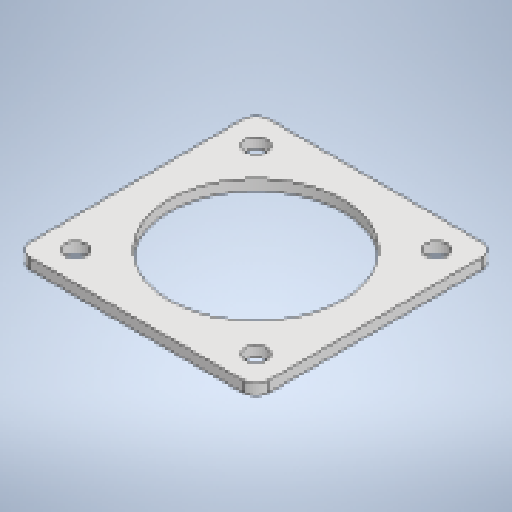
# Autodesk Inventor part: NDM-VOS 162 harrow plate 5
Saved by Autodesk Inventor 2025.1 (Build 291241020, 241B)
## iProperties
Created: 2024-11-03
Part Number: NDM-VOS 162 harrow plate 5
Material: Stainless Steel
Document SubType Name: Sheet Metal
Designer: user
Mass: 280.619 g
Surface Area: 364.406 cm^2
Volume: 35.0774 cm^3
Density: 8 g/cm^3
Sheet Metal Rule: AISI304 3mm Die 32
Sheet Metal Width: 0,000 mm
Sheet Metal Length: 0,000 mm
Sheet Metal Area: 0,000 mm^2
Appearance: Default
Author: admin
Гриндер_отступ_отврс_корпуса: 25.000 mm
Гриндер_диам_отврс_корпуса: 13.000 mm
Гриндер_проходная_ширина: 320.000 mm
Гриндер_проходная_длина: 320.000 mm
Гриндер_высота: 200.000 mm
Гриндер_размер_фланца: 40.000 mm
Гриндер_Валы_между_центрами: 150.000 mm
Autodesk Inventor part; units mm, degrees
ref_plane "YZ Plane" through (0, 0, 0) normal (1, 0, 0) x (0, 1, 0)
ref_plane "XZ Plane" through (0, 0, 0) normal (0, 1, 0) x (-1, 0, 0)
ref_plane "XY Plane" through (0, 0, 0) normal (0, 0, 1) x (1, 0, 0)
sketch "Sketch1" plane through (0, 0, 0) normal (0, 0, 1) x (1, 0, 0)
  line L0 (-200, 100) -> (200, 100)
  line L1 (200, 100) -> (200, -100)
  line L2 (200, -100) -> (-200, -100)
  line L3 (-200, -100) -> (-200, 100)
  line L4 (-200, 100) -> (200, -100) construction
  line L5 (200, 100) -> (-200, -100) construction
  point P0 (0, 0)
  point P1 (0, 0)
  point P2 (0, 0)
  dimension "d25" = 400
  dimension "d26" = 200
  measures "d25" distance of L1.end L2.end
  measures "d26" distance of L0.end L1.end
extrude "Plate1" add sketch "Sketch1" along normal blind 5
sketch "Sketch5" plane through (-195, -100, 0) normal (-1, 0, 0) x (0, -1, 0)
  line L0 (-200, 0) -> (0, 0)
  line L1 (0, 0) -> (0, 50)
  line L2 (0, 50) -> (-200, 50)
  line L3 (-200, 50) -> (-200, 0)
  constraints: 6 end point, 1 horizontal, 1 perpendicular, 1 vertical
edge flange "Flange2" height 50 angle 90 thickness 5 bend radius 5 thickness toward (-1, 0, 0) relief round relief width 5 relief depth 2.5 corner gap 5 corner form 0 edges at (-200, 0, 5) (200, 0, 5) (0, 100, 5) (0, -100, 5) wall of the first edge with corners at (-195, 100, 0) (-195, -100, 0) (-195, -100, 50) (-195, 100, 50)
bend "Bend2"
corner "Corner2"
sketch "Sketch6" plane through (0, 0, 5) normal (0, 0, 1) x (1, 0, 0)
  circle A0 centre (-75, 0) radius 16
  circle A1 centre (75, 0) radius 16
  line L0 (0, 0) -> (0, 55.0725) construction
  circle A2 centre (33.5, 41.5) radius 5
  circle A3 centre (116.5, 41.5) radius 5
  circle A4 centre (116.5, -41.5) radius 5
  circle A5 centre (33.5, -41.5) radius 5
  line L1 (75, 0) -> (-75, 0)
  line L2 (75, 0) -> (75, -40.8866)
  circle A6 centre (-33.5, 41.5) radius 5
  circle A7 centre (-116.5, 41.5) radius 5
  circle A8 centre (-116.5, -41.5) radius 5
  circle A9 centre (-33.5, -41.5) radius 5
  point P0 (-75, -40.8866)
  dimension "d37" = 32
  dimension "d38" = 150
  dimension "d55" = 10
  dimension "d56" = 83
  dimension "d57" = 83
  constraints: 10 centre point, 8 symmetric about line, 6 end point, 3 equal radius, 3 horizontal alignment, 2 vertical, 2 vertical alignment, 1 horizontal, 5 other
  measures "d37" diameter of A0
  measures "d38" distance of L1.start L1.end
  measures "d55" diameter of A3
  measures "d56" distance of A3.centre A2.centre
  measures "d57" distance of A4.centre A3.centre
extrude "Cut1" cut sketch "Sketch6" against normal blind 5
sketch "Sketch7" plane through (-194.2929, 100, 10) normal (0, 1, 0) x (1, 0, 0)
  circle A0 centre (194.2929, -20) radius 6.5
  line L0 (5, 5) -> (383.5858, 5) projected
  line L1 (383.5858, 5) -> (384.2929, 5) projected
  line L2 (384.2929, 5) -> (383.5858, 5) projected
  line L3 (383.5858, 5) -> (5, 5) projected
  line L4 (5, 5) -> (4.2929, 5) projected
  line L5 (4.2929, 5) -> (5, 5) projected
  point P0 (194.2929, 10)
  dimension "d41" = 13
  dimension "d42" = 25
  constraints: 1 centre point, 1 vertical alignment
  measures "d41" diameter of A0
  measures "d42" distance from line of A0.centre L0
extrude "Extrusion2" cut sketch "Sketch7" against normal through all
pattern_linear "Rectangular Pattern1" count 3 spacing 160 along (-1, 0, 0) of "Extrusion2" first direction both ways yes
sketch "Sketch8" plane through (0, 0, 0) normal (1, 0, 0) x (0, 1, 0)
  line L0 (-94.2929, 50) -> (94.2929, 50) projected
  circle A0 centre (0, 30) radius 6.5
  line L1 (89.2929, 5) -> (-89.2929, 5) projected
  point P0 (0, 0)
  dimension "d48" = 13
  dimension "d49" = 25
  constraints: 1 centre point, 1 vertical alignment
  measures "d48" diameter of A0
  measures "d49" distance from line of L1 A0.centre
extrude "Extrusion3" cut sketch "Sketch8" along normal through all both and the other way through all
pattern_linear "Rectangular Pattern2" count 3 spacing 70 along (0, 1, 0) of "Extrusion3" first direction both ways yes
sketch "Sketch9" plane through (0, 0, 0) normal (0, 0, 1) x (1, 0, 0)
  line L0 (-233.1694, -164.5287) -> (298.5547, -164.5287)
  line L1 (298.5547, -164.5287) -> (298.5547, 258.31)
  line L2 (298.5547, 258.31) -> (-233.1694, 258.31)
  line L3 (-233.1694, 258.31) -> (-233.1694, -164.5287)
  circle A0 centre (-75, 0) radius 16 projected
  line L4 (-130, -55) -> (-20, -55)
  line L5 (-20, -55) -> (-20, 55)
  line L6 (-20, 55) -> (-130, 55)
  line L7 (-130, 55) -> (-130, -55)
  line L8 (-130, -55) -> (-20, 55) construction
  line L9 (-20, -55) -> (-130, 55) construction
  circle A1 centre (-75, 0) radius 40
  point P0 (0, 0)
  dimension "d58" = 110
  dimension "d59" = 110
  dimension "d60" = 80
  constraints: 20 end point, 4 parallel, 2 horizontal, 2 midpoint, 2 perpendicular, 1 centre point, 1 coincident
  measures "d58" distance of L6.end L5.end
  measures "d59" distance of L5.end L4.end
  measures "d60" diameter of A1
extrude "Extrusion4" cut sketch "Sketch9" along normal through all both and the other way through all
fillet "Corner Round1" radius 6 4 edges at (-130, -55, 2.5) (-130, 55, 2.5) (-20, 55, 2.5) (-20, -55, 2.5)
equation "\"d25\" = Гриндер_проходная_ширина + 2 * Гриндер_размер_фланца"
equation "\"d26\" = Гриндер_высота"
equation "\"d38\" = Гриндер_Валы_между_центрами"
equation "\"d57\" = d56"
equation "\"d39\" = Thickness"
equation "\"d41\" = Гриндер_диам_отврс_корпуса"
equation "\"d42\" = Гриндер_отступ_отврс_корпуса"
equation "\"d48\" = Гриндер_диам_отврс_корпуса"
equation "\"d49\" = Гриндер_отступ_отврс_корпуса"
equation "\"d2\" = Thickness"
equation "\"d27\" = BendReliefWidth"
equation "\"d28\" = BendReliefDepth"
equation "\"d29\" = MinimumRemnant"
equation "\"d30\" = TransitionRadius"
equation "\"d33\" = BendRadius"
equation "\"d34\" = CornerReliefSize"
equation "\"d36\" = JacobiRadiusSize"
equation "\"BendReliefWidth\" = Thickness"
equation "\"BendReliefDepth\" = 0.5 * Thickness"
equation "\"TransitionRadius\" = BendRadius"
equation "\"JacobiRadiusSize\" = BendRadius"
equation "\"GapSize\" = Thickness"
equation "\"Гриндер_отступ_отврс_корпуса\" = 25"
equation "\"Гриндер_диам_отврс_корпуса\" = 13"
equation "\"Гриндер_проходная_ширина\" = 320"
equation "\"Гриндер_проходная_длина\" = 320"
equation "\"Гриндер_высота\" = 200"
equation "\"Гриндер_размер_фланца\" = 40"
equation "\"Гриндер_Валы_между_центрами\" = 150"
equation "\"Thickness\" = 5"
equation "\"MinimumRemnant\" = 10"
equation "\"BendRadius\" = 5"
equation "\"CornerReliefSize\" = 20"
body "Solid1"
